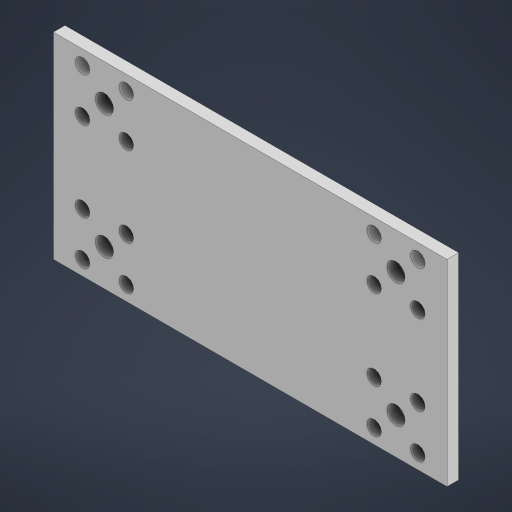
# Autodesk Inventor part: TurretMotorPlate
Saved by Autodesk Inventor 2024 (Build 280153000, 153)
## iProperties
Created: 2023-10-20
Part Number: TurretMotorPlate
Material: Generic
Document SubType Name: Modeling
Designer: avsar
Density: 1 g/cm^3
Appearance: Default
Author: avsar
Autodesk Inventor part; units mm, degrees
ref_plane "YZ Plane" through (0, 0, 0) normal (1, 0, 0) x (0, 1, 0)
ref_plane "XZ Plane" through (0, 0, 0) normal (0, 1, 0) x (-1, 0, 0)
ref_plane "XY Plane" through (0, 0, 0) normal (0, 0, 1) x (1, 0, 0)
sketch "Sketch1" plane through (0, 0, 0) normal (0, 0, 1) x (1, 0, 0)
  line L0 (-54, -27) -> (54, -27)
  line L1 (54, -27) -> (54, 27)
  line L2 (54, 27) -> (-54, 27)
  line L3 (-54, 27) -> (-54, -27)
  line L4 (-54, -27) -> (54, 27) construction
  line L5 (54, -27) -> (-54, 27) construction
  point P0 (0, 0)
  dimension "d0" = 108
  dimension "d1" = 54
  constraints: 12 end point, 2 midpoint, 2 parallel, 1 horizontal, 1 perpendicular
  measures "d0" distance of L2.end L1.end
  measures "d1" distance of L1.end L0.end
extrude "Extrusion1" add sketch "Sketch1" along normal blind 3.175
sketch "Sketch2" plane through (0, 0, 3.175) normal (0, 0, 1) x (1, 0, 0)
  line L0 (-54, -27) -> (54, -27) construction
  line L1 (54, -27) -> (54, 27) construction
  line L2 (54, 27) -> (-54, 27) construction
  line L3 (-54, 27) -> (-54, -27) construction
  line L4 (-54, -27) -> (54, -27) projected
  line L5 (0, 27) -> (0, -27) construction
  circle A0 centre (-40, -17) radius 2.5
  circle A1 centre (-46, -23) radius 2
  circle A2 centre (-34, -23) radius 2
  circle A3 centre (-34, -11) radius 2
  circle A4 centre (-46, -11) radius 2
  circle A5 centre (40, -17) radius 2.5
  circle A6 centre (46, -23) radius 2
  circle A7 centre (34, -23) radius 2
  circle A8 centre (34, -11) radius 2
  circle A9 centre (46, -11) radius 2
  line L6 (-54, 0) -> (54, 0) construction
  circle A10 centre (-40, 17) radius 2.5
  circle A11 centre (-46, 23) radius 2
  circle A12 centre (-34, 23) radius 2
  circle A13 centre (-34, 11) radius 2
  circle A14 centre (-46, 11) radius 2
  circle A15 centre (34, 11) radius 2
  circle A16 centre (34, 23) radius 2
  circle A17 centre (40, 17) radius 2.5
  circle A18 centre (46, 11) radius 2
  circle A19 centre (46, 23) radius 2
  point P0 (0, 0)
  point P1 (0, 0)
  point P2 (0, 0)
  dimension "d11" = 5
  dimension "d12" = 40
  dimension "d13" = 10
  dimension "d14" = 4
  dimension "d15" = 6
  dimension "d16" = 6
  dimension "d19" = 360
  constraints: 20 centre point, 15 symmetric about line, 6 midpoint, 4 end point, 24 other
  measures "d11" diameter of A0
  measures "d12" horizontal distance of point (0, 0) A0.centre
  measures "d13" distance from line of L0 A0.centre
  measures "d14" diameter of A1
  measures "d15" horizontal distance of A0.centre A1.centre
  measures "d16" horizontal distance of A0.centre A1.centre
extrude "Extrusion2" cut sketch "Sketch2" against normal through all
body "Solid1"
